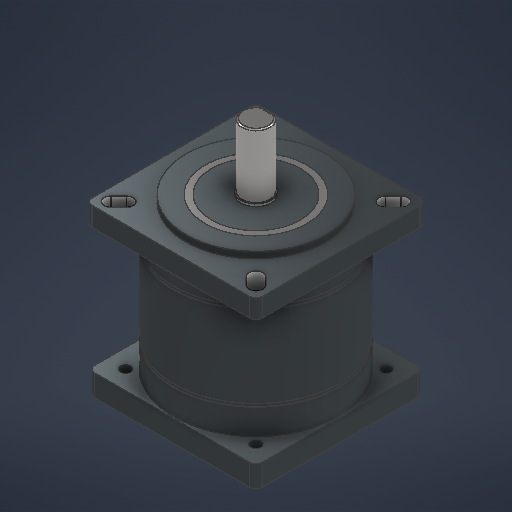
# Autodesk Inventor part: PX130-GEARBOX
Saved by Autodesk Inventor 2025.3 (Build 293356030, 356C)
## iProperties
Created: 2025-10-20
Part Number: PX130-GEARBOX
Material: Generic
Document SubType Name: Modeling
Designer: lstk1ng
Density: 4.37701 g/cm^3
Appearance: Default
Mass: 8100 g
Surface Area: 1167.79 cm^2
Volume: 1850.58 cm^3
Author: lstk1ng
Autodesk Inventor part; units mm, degrees
ref_plane "YZ Plane" through (0, 0, 0) normal (1, 0, 0) x (0, 1, 0)
ref_plane "XZ Plane" through (0, 0, 0) normal (0, 1, 0) x (-1, 0, 0)
ref_plane "XY Plane" through (0, 0, 0) normal (0, 0, 1) x (1, 0, 0)
sketch "Sketch1" plane through (0, 0, 0) normal (0, 1, 0) x (-1, 0, 0)
  line L0 (-61, 66) -> (61, 66)
  line L1 (66, 61) -> (66, -61)
  line L2 (61, -66) -> (-61, -66)
  line L3 (-66, -61) -> (-66, 61)
  line L4 (-66, 66) -> (66, -66) construction
  line L5 (66, 66) -> (-66, -66) construction
  circle A0 centre (0, 0) radius 72.5 construction
  circle A1 centre (51.2652, 51.2652) radius 4
  circle A2 centre (51.2652, -51.2652) radius 4
  line L6 (0, 66) -> (0, 0) construction
  circle A3 centre (-51.2652, 51.2652) radius 4
  circle A4 centre (-51.2652, -51.2652) radius 4
  arc A5 (61, -66) -> (66, -61) centre (61, -61) ccw
  arc A6 (-66, -61) -> (-61, -66) centre (-61, -61) ccw
  line L7 (0, 0) -> (66, 0) construction
  arc A7 (66, 61) -> (61, 66) centre (61, 61) ccw
  arc A8 (-61, 66) -> (-66, 61) centre (-61, 61) ccw
  dimension "d0" = 132
  dimension "d1" = 132
  dimension "d3" = 8
  dimension "d4" = 8
  dimension "d5" = 5
  dimension "d47" = 145
  constraints: 16 end point, 10 point on circle, 9 centre point, 8 symmetric about line, 6 point on line, 4 midpoint, 4 tangent, 2 parallel, 2 perpendicular, 1 coincident, 1 equal radius, 1 horizontal, 1 vertical, 4 other
  measures "d0" distance of L4.end L5.end
  measures "d1" distance of L5.start L4.end
  measures "d3" diameter of A1
  measures "d4" diameter of A2
  measures "d5" radius of A5
  measures "d47" diameter of A0
extrude "Extrusion1" add sketch "Sketch1" along normal blind 17
sketch "Sketch2" plane through (0, 17, 0) normal (0, 1, 0) x (1, 0, 0)
  circle A0 centre (0, 0) radius 65
  dimension "d8" = 130
  constraints: 1 centre point, 1 coincident
  measures "d8" diameter of A0
extrude "Extrusion2" add sketch "Sketch2" along normal blind 99
sketch "Sketch3" plane through (0, 116, 0) normal (0, 1, 0) x (1, 0, 0)
  line L0 (62, 67) -> (-62, 67)
  line L1 (-67, 62) -> (-67, -62)
  line L2 (-62, -67) -> (62, -67)
  line L3 (67, -62) -> (67, 62)
  line L4 (-67, 67) -> (67, -67) construction
  arc A0 (-67, -62) -> (-62, -67) centre (-62, -62) ccw
  arc A1 (-62, 67) -> (-67, 62) centre (-62, 62) ccw
  arc A2 (67, 62) -> (62, 67) centre (62, 62) ccw
  arc A3 (62, -67) -> (67, -62) centre (62, -62) ccw
  line L5 (51, -51) -> (-51, -51) construction
  line L6 (-51, -51) -> (-51, 51) construction
  line L7 (-51, 51) -> (51, 51) construction
  line L8 (51, 51) -> (51, -51) construction
  line L9 (51, -51) -> (-51, 51) construction
  line L10 (-51, -51) -> (51, 51) construction
  line L11 (57, -57) -> (-57, -57) construction
  line L12 (-57, -57) -> (-57, 57) construction
  line L13 (-57, 57) -> (57, 57) construction
  line L14 (57, 57) -> (57, -57) construction
  line L15 (-57, -57) -> (-51, -51) construction
  line L16 (0, 0) -> (0, 51) construction
  line L17 (0, 0) -> (51, 0) construction
  line L18 (-54, -54) -> (-47.1057, -47.1057) construction
  line L19 (-51, -51) -> (-57, -57) construction
  line L20 (-54.8943, -47.1057) -> (-60.8943, -53.1057)
  line L21 (-53.1057, -60.8943) -> (-47.1057, -54.8943)
  arc A4 (-47.1057, -54.8943) -> (-54.8943, -47.1057) centre (-51, -51) ccw
  arc A5 (-60.8943, -53.1057) -> (-53.1057, -60.8943) centre (-57, -57) ccw
  line L22 (51, -51) -> (54, -54) construction
  line L23 (54, -54) -> (47.1057, -47.1057) construction
  line L24 (51, -51) -> (57, -57) construction
  line L25 (47.1057, -54.8943) -> (53.1057, -60.8943)
  line L26 (60.8943, -53.1057) -> (54.8943, -47.1057)
  arc A6 (54.8943, -47.1057) -> (47.1057, -54.8943) centre (51, -51) ccw
  arc A7 (53.1057, -60.8943) -> (60.8943, -53.1057) centre (57, -57) ccw
  line L27 (51, 51) -> (54, 54) construction
  line L28 (54, 54) -> (47.1057, 47.1057) construction
  line L29 (51, 51) -> (57, 57) construction
  line L30 (54.8943, 47.1057) -> (60.8943, 53.1057)
  line L31 (53.1057, 60.8943) -> (47.1057, 54.8943)
  arc A8 (47.1057, 54.8943) -> (54.8943, 47.1057) centre (51, 51) ccw
  arc A9 (60.8943, 53.1057) -> (53.1057, 60.8943) centre (57, 57) ccw
  line L32 (-51, 51) -> (-57, 57) construction
  line L33 (-51, 51) -> (-54, 54) construction
  line L34 (-54, 54) -> (-47.1057, 47.1057) construction
  line L35 (-51, 51) -> (-57, 57) construction
  line L36 (-47.1057, 54.8943) -> (-53.1057, 60.8943)
  line L37 (-60.8943, 53.1057) -> (-54.8943, 47.1057)
  arc A10 (-54.8943, 47.1057) -> (-47.1057, 54.8943) centre (-51, 51) ccw
  arc A11 (-53.1057, 60.8943) -> (-60.8943, 53.1057) centre (-57, 57) ccw
  point P0 (-67, 0)
  point P1 (0, 67)
  dimension "d22" = 5
  dimension "d48" = 102
  dimension "d49" = 102
  dimension "d50" = 114
  dimension "d51" = 114
  dimension "d53" = 9.75
  dimension "d76" = 9.75
  dimension "d77" = 9.75
  dimension "d78" = 9.75
  constraints: 86 end point, 24 point on circle, 24 tangent, 13 midpoint, 12 centre point, 10 parallel, 9 point on line, 4 collinear, 3 equal radius, 3 horizontal, 3 perpendicular, 1 horizontal alignment, 1 vertical alignment
  measures "d22" radius of A0
  measures "d48" distance of L6.end L7.end
  measures "d49" distance of L5.end L6.end
  measures "d50" distance of L12.end L13.end
  measures "d51" distance of L11.end L12.end
  measures "d53" distance of L18.start L18.end
  measures "d76" distance of L22.end L23.end
  measures "d77" distance of L27.end L28.end
  measures "d78" distance of L33.end L34.end
extrude "Extrusion3" add sketch "Sketch3" along normal blind 15
sketch "Sketch4" plane through (0, 131, 0) normal (0, 1, 0) x (1, 0, 0)
  circle A0 centre (0, 0) radius 55
  dimension "d19" = 110
  constraints: 1 centre point, 1 coincident
  measures "d19" diameter of A0
extrude "Extrusion4" add sketch "Sketch4" along normal blind 5
sketch "Sketch5" plane through (0, 136, 0) normal (0, 1, 0) x (1, 0, 0)
  arc A0 (-3, 10.583) -> (3, 10.583) centre (0, 0) ccw
  line L0 (0, -11) -> (0, 13.5) construction
  line L1 (-3, 8.5) -> (3, 8.5)
  line L2 (3, 8.5) -> (3, 10.583)
  line L3 (-3, 10.583) -> (-3, 8.5)
  line L4 (-3, 8.5) -> (3, 13.5) construction
  line L5 (3, 8.5) -> (-3, 13.5) construction
  dimension "d54" = 22
  constraints: 12 end point, 3 point on circle, 1 centre point, 1 horizontal, 1 parallel, 1 perpendicular, 1 vertical
  measures "d54" diameter of A0
extrude "Extrusion5" add sketch "Sketch5" along normal blind 52
sketch "Sketch7" plane through (0, 0, 0) normal (0, 0, 1) x (1, 0, 0)
  line L0 (-65, 106) -> (-65, 103.5)
  line L1 (-65, 106) -> (-64.5, 106)
  line L2 (-64.5, 106) -> (-64.5, 103.5)
  line L3 (-64.5, 103.5) -> (-65, 103.5)
  line L4 (-65, 17) -> (-65, 37) construction
  line L5 (-65, 37) -> (-64.5, 37)
  line L6 (-64.5, 37) -> (-64.5, 39.5)
  line L7 (-64.5, 39.5) -> (-65, 39.5)
  line L8 (-65, 39.5) -> (-65, 37)
  line L9 (0, -27.2) -> (0, 163.2) projected
  line L10 (-65, 121) -> (-65, 106) construction
  point P0 (0, 0)
  dimension "d35" = 2.5
  dimension "d36" = 0.5
  dimension "d37" = 20
  dimension "d38" = 0.5
  dimension "d39" = 2.5
  dimension "d41" = 15
  constraints: 20 end point, 4 perpendicular, 2 horizontal, 1 vertical
  measures "d35" distance of L0.start L0.end
  measures "d36" distance of L0.start L1.end
  measures "d37" distance of L4.start L4.end
  measures "d38" distance of L4.end L5.end
  measures "d39" distance of L5.end L6.end
  measures "d41" distance of L10.start L10.end
revolve "Revolution1" cut sketch "Sketch7" angle 360 about axis through (0, -10, 0) along (0, 1, 0)
sketch "Sketch8" plane through (0, 0, 0) normal (0, -1, 0) x (1, 0, 0)
  arc A0 (-3, 10.583) -> (3, 10.583) centre (0, 0) ccw
  line L0 (0, -11) -> (0, 13.7) construction
  line L1 (3, 10.583) -> (3, 13.7)
  line L2 (3, 13.7) -> (-3, 13.7)
  line L3 (-3, 13.7) -> (-3, 10.583)
  line L4 (-3, 8.3) -> (3, 13.7) construction
  line L5 (3, 8.3) -> (-3, 13.7) construction
  dimension "d72" = 22
  dimension "d73" = 24.7
  dimension "d74" = 6
  constraints: 12 end point, 3 point on circle, 1 centre point, 1 parallel, 1 vertical
  measures "d72" diameter of A0
  measures "d73" distance of L0.start L0.end
  measures "d74" distance of L2.end L1.end
extrude "Extrusion7" cut sketch "Sketch8" against normal blind 62
sketch "Sketch11" plane through (0, 136, 0) normal (0, 1, 0) x (1, 0, 0)
  circle A0 centre (0, 0) radius 12
  dimension "d60" = 24
  constraints: 1 centre point, 1 coincident
  measures "d60" diameter of A0
extrude "Extrusion9" add sketch "Sketch11" along normal blind 2
chamfer "Chamfer1" distance 1 angle 45 1 edges at (0, 188, 11)
sketch "Sketch12" plane through (0, 136, 0) normal (0, 1, 0) x (1, 0, 0)
  circle A0 centre (0, 0) radius 35
  circle A1 centre (0, 0) radius 40
  dimension "d66" = 70
  constraints: 2 centre point, 1 coincident
  measures "d66" diameter of A0
extrude "Extrusion10" cut sketch "Sketch12" against normal blind 0.0001
sketch "Sketch13" plane through (0, 0, 0) normal (0, -1, 0) x (1, 0, 0)
  circle A0 centre (0, 0) radius 55
  dimension "d69" = 110
  constraints: 1 centre point, 1 coincident
  measures "d69" diameter of A0
extrude "Extrusion11" cut sketch "Sketch13" against normal blind 6
body "Solid1"
